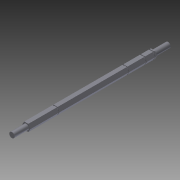
# Autodesk Inventor part: 0.5 in Hex Shaft V3
Saved by Autodesk Inventor 2014 SP1 (Build 180222100, 222)
## iProperties
Created: 2012-01-16
Part Number: 0.5 in Hex Shaft V3
Material: Steel
Document SubType Name: Modeling
Designer: Moses
Density: 7.85 g/cm^3
Mass: 276.089 g
Surface Area: 121.09 cm^2
Volume: 35.1706 cm^3
Appearance: Steel
Author: Moses
Autodesk Inventor part; units mm, degrees
ref_plane "YZ Plane" through (0, 0, 0) normal (1, 0, 0) x (0, 1, 0)
sketch "Sketch1" plane through (0, 0, 0) normal (0, 0, 1) x (1, 0, 0)
  line L0 (7.3323, 0) -> (3.6662, -6.35)
  line L1 (3.6662, -6.35) -> (-3.6662, -6.35)
  line L2 (-3.6662, -6.35) -> (-7.3323, 0)
  line L3 (-7.3323, 0) -> (-3.6662, 6.35)
  line L4 (-3.6662, 6.35) -> (3.6662, 6.35)
  line L5 (3.6662, 6.35) -> (7.3323, 0)
  point P0 (0, 0)
  point P1 (0, 0)
  dimension "d0" = 12.7
  constraints: 12 end point, 1 coincident, 1 horizontal, 13 other
  measures "d0" distance between parallel lines of L1 L4
extrude "Extrusion1" add sketch "Sketch1" along normal blind 114.3
sketch "Sketch2" plane through (0, 0, 114.3) normal (0, 0, 1) x (1, 0, 0)
  circle A0 centre (0, 0) radius 4.7625
  dimension "d3" = 9.525
  constraints: 1 centre point, 1 coincident
  measures "d3" diameter of A0
extrude "Extrusion2" add sketch "Sketch2" along normal blind 25.4
mirror "Mirror1" about plane through (0, 0, 0) normal (0, 0, -1) of "Extrusion2", "Extrusion1"
ref_plane "Work Plane1" through (1.8331, 3.175, -114.3) normal (-0.8660254, 0.5, 0) x (0, 0, 1)
sketch "Sketch3" plane through (1.8331, 3.175, -114.3) normal (-0.8660254, 0.5, 0) x (0, 0, 1)
  line L0 (-25.4, 1.0963) -> (-25.4, -8.4287) construction
  line L1 (0, 1.0963) -> (0, -8.4287) construction
  line L2 (-25.4, 1.0963) -> (0, 1.0963) construction
  line L3 (-25.4, -8.4287) -> (0, -8.4287) construction
  line L4 (228.6, 3.6662) -> (0, 3.6662) construction
  line L5 (228.6, -7.3323) -> (228.6, 0) construction
  line L6 (228.6, 0) -> (0, 0) construction
  line L7 (0, -7.3323) -> (0, 0) construction
  line L8 (228.6, -7.3323) -> (0, -7.3323) construction
  line L9 (228.6, 0) -> (228.6, 3.6662) construction
  line L10 (228.6, 3.6662) -> (0, 3.6662) construction
  line L11 (0, 0) -> (0, 3.6662) construction
  line L12 (228.6, 0) -> (0, 0) construction
  line L13 (228.6, -10.9985) -> (228.6, -7.3323) construction
  line L14 (228.6, -7.3323) -> (0, -7.3323) construction
  line L15 (0, -10.9985) -> (0, -7.3323) construction
  line L16 (228.6, -10.9985) -> (0, -10.9985) construction
  line L17 (254, 1.0963) -> (254, -8.4287) construction
  line L18 (228.6, 1.0963) -> (228.6, -8.4287) construction
  line L19 (228.6, 1.0963) -> (254, 1.0963) construction
  line L20 (228.6, -8.4287) -> (254, -8.4287) construction
  line L21 (-25.4, -3.6662) -> (254, -3.6662) construction
  line L22 (3.81, 14.6218) -> (3.81, 1.9218)
  line L23 (3.81, 1.9218) -> (5.334, 1.9218)
  line L24 (5.334, 1.9218) -> (5.334, 14.6218)
  line L25 (5.334, 14.6218) -> (3.81, 14.6218)
  line L26 (19.6342, 14.6218) -> (19.6342, 1.9218)
  line L27 (19.6342, 1.9218) -> (21.1582, 1.9218)
  line L28 (21.1582, 1.9218) -> (21.1582, 14.6218)
  line L29 (21.1582, 14.6218) -> (19.6342, 14.6218)
  line L30 (0, 1.9218) -> (228.6, 1.9218) construction
  line L31 (51.054, 1.9218) -> (51.054, 14.6218)
  line L32 (51.054, 14.6218) -> (52.578, 14.6218)
  line L33 (52.578, 14.6218) -> (52.578, 1.9218)
  line L34 (51.054, 1.9218) -> (52.578, 1.9218)
  line L35 (176.022, 1.9218) -> (176.022, 14.6218)
  line L36 (176.022, 14.6218) -> (177.546, 14.6218)
  line L37 (177.546, 14.6218) -> (177.546, 1.9218)
  line L38 (176.022, 1.9218) -> (177.546, 1.9218)
  line L39 (0, 13.7963) -> (0, 1.0963)
  line L40 (0, 1.0963) -> (1.6002, 1.0963)
  line L41 (1.6002, 1.0963) -> (1.6002, 13.7963)
  line L42 (1.6002, 13.7963) -> (0, 13.7963)
  line L43 (228.346, 13.7963) -> (228.346, 1.0963)
  line L44 (228.346, 1.0963) -> (228.6, 1.0963)
  line L45 (228.6, 1.0963) -> (228.6, 13.7963)
  line L46 (228.6, 13.7963) -> (228.346, 13.7963)
  point P0 (114.3, -3.6662)
  dimension "d6" = 12.7
  dimension "d7" = 1.524
  dimension "d10" = 1.524
  dimension "d11" = 5.588
  dimension "d13" = 1.524
  dimension "d14" = 1.524
  dimension "d16" = 14.3002
  dimension "d18" = 123.444
  dimension "d19" = 61.722
  dimension "d23" = 1.6002
  dimension "d24" = 12.7
  dimension "d25" = 12.7
  dimension "d26" = 0.254
  dimension "d27" = 3.81
  constraints: 52 end point, 15 perpendicular, 12 parallel, 12 point on line, 2 midpoint, 1 collinear
  measures "d6" distance of L23.end L24.end
  measures "d7" distance of L24.end L22.start
  measures "d10" distance of L28.end L26.start
  measures "d11" distance between parallel lines of L21 L30
  measures "d13" distance of L31.end L32.end
  measures "d14" distance of L35.end L36.end
  measures "d16" distance between parallel lines of L26 L24
  measures "d18" distance between parallel lines of L35 L33
  measures "d19" distance from line of point (114.3, -3.666) L33
  measures "d23" distance of L39.end L40.end
  measures "d24" distance of L39.start L39.end
  measures "d25" distance of L43.start L43.end
  measures "d26" distance of L45.end L43.start
  measures "d27" distance between parallel lines of L1 L22
revolve "Revolution1" cut sketch "Sketch3" angle 360 about axis through (0, 0, -139.7) along (0, 0, 1)
ref_plane "Work Plane2" through (-3.6662, -6.35, 0) normal (0, 0, 1) x (1, 0, 0)
equation "\"d10\" = d7"
equation "\"d13\" = d7"
equation "\"d14\" = d7"
equation "\"d19\" = 0.5 * d18"
equation "\"d25\" = d6"
body "Solid1"
